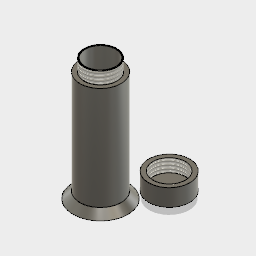
水杯 vip (Autodesk Fusion 360 design; units mm, degrees)
Autodesk Fusion 360 part; units mm, degrees
cylinder "圆柱体基本要素1" add diameter 60 height 150 placed x (1, 0, 0) y (0, 0, -1) z (0, 1, 0) at (0, 0, 0) makes body 1
shell "抽壳1" thickness 8 removed faces 1 at (7.6631, 150, -11.2397) on bodies 1
cylinder "圆柱体基本要素2" add diameter 48 height 18 placed x (1, 0, 0) y (0, 0, -1) z (0, 1, 0) at (0, 150, 0) bodies 1
sketch "草图6" plane through (0, 168, 0) normal (0, 1, 0) x (-1, 0, 0)
  circle A0 centre (0, 0) radius 24
  circle A1 centre (0, 0) radius 22
  dimension "d6" = 44
  measures "d6" diameter of A1
extrude "拉伸1" cut sketch "草图6" against normal blind 18 contours A1 bodies 1
thread "螺纹1" "ISO Metric profile 48.0 M48x5 6g" major diameter 47.664 minor diameter 41.9335 pitch 5 angle 60 resizes the face on face at (23.8807, 162, 2.3896) from (0, 151, 0) to (0, 168, 0) on bodies 1
fillet "圆角1" radius 0.6 1 edges at (20.5112, 168, 7.9555) on bodies 1
fillet "圆角2" radius 0.6 1 edges at (-22.2192, 168, 8.618) on bodies 1
cylinder "圆柱体基本要素3" add diameter 60 height 25 placed x (1, 0, 0) y (0, 0, -1) z (0, 1, 0) at (50, 0, -50) separate body makes body 2
shell "抽壳2" thickness 6 removed faces 1 at (44.6674, 25, -63.0982) on bodies 2
thread "螺纹2" "ISO Metric profile 52.0 M52x5 6H" major diameter 52.5183 minor diameter 46.9423 pitch 5 angle 60 resizes the face on face at (73.8807, 12.3333, -47.6104) on bodies 2
sketch "草图8" plane through (0, 0, 0) normal (0, 1, 0) x (1, 0, 0)
  arc A0 (150, -25) -> (125, 0) centre (127.2881, -22.7119) ccw
  arc A1 (140, -30) -> (123.7537, -8.9729) centre (125.7186, -24.2445) ccw
  line L0 (125, 0) -> (123.7537, -8.9729)
  line L1 (150, -25) -> (140, -30)
extrude "拉伸2" add sketch "草图8" along normal blind 10 separate body makes body 3
move_body "移动1" bodies 3 to x (1, 0, 0) y (0, 1, 0) z (0, 0, 1) at (-210.0534, 0, -142.8836)
move_body "移动2" bodies 3 to x (0.573576, 0, -0.819152) y (0, 1, 0) z (0.819152, 0, 0.573576) at (141.4733, -1.7814, -10.6116)
move_body "移动3" bodies 3 to x (1, 0, 0) y (0, 1, 0) z (0, 0, 1) at (0, 40, 0)
move_body "移动4" bodies 3 to x (1, 0, 0) y (0, 1, 0) z (0, 0, 1) at (3, 0, 3)
move_body "移动5" bodies 3 to x (1, 0, 0) y (0, 1, 0) z (0, 0, 1) at (0, 30, 0)
sketch "草图9" plane through (0, 0, 0) normal (0, 1, 0) x (1, 0, 0)
  circle A0 centre (60, -40) radius 30
  circle A1 through (100, -40, -10) (40, -5.359, -10) (40, -74.641, -10)
loft "放样1" add profiles "草图9", "草图9" section 1 section 2 contours A1 in plane through (0, -10, 0) normal (0, 1, 0) separate body makes body 4
move_body "移动6" bodies 4 to x (1, 0, 0) y (0, 0.819152, -0.573576) z (0, 0.573576, 0.819152) at (-11.6211, -13.4785, 37.3424)
shell "抽壳3" thickness 1 removed faces 1 at (36.437, 1.0268, 75.4927) on bodies 4
move_body "对齐1" bodies 4 to x (1, 0, 0) y (0, 0.819152, 0.573576) z (0, -0.573576, 0.819152) at (-48.3789, 32.4597, -62.8581)
combine "合并1" operation add target body 1 tool bodies 4
